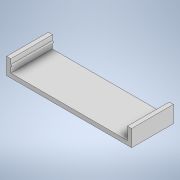
# Autodesk Inventor part: Houderpi
Saved by Autodesk Inventor 2021 (Build 250183000, 183)
## iProperties
Created: 2023-11-14
Part Number: Houderpi
Material: Generic
Document SubType Name: Modeling
Designer: Elias
Density: 1 g/cm^3
Appearance: Default
Author: Elias
Autodesk Inventor part; units mm, degrees
ref_plane "YZ Plane" through (0, 0, 0) normal (1, 0, 0) x (0, 1, 0)
ref_plane "XZ Plane" through (0, 0, 0) normal (0, 1, 0) x (-1, 0, 0)
ref_plane "XY Plane" through (0, 0, 0) normal (0, 0, 1) x (1, 0, 0)
sketch "Sketch1" plane through (0, 0, 0) normal (0, 0, 1) x (1, 0, 0)
  line L0 (0, 0) -> (60, 0)
  line L1 (60, 0) -> (60, 8)
  line L2 (60, 8) -> (0, 8)
  line L3 (0, 8) -> (0, 0)
  dimension "d0" = 60
  dimension "d3" = 8
  constraints: 8 end point, 2 parallel, 1 horizontal, 1 perpendicular
  measures "d0" distance of L2.end L1.end
  measures "d3" distance of L0.end L1.end
extrude "Extrusion1" add sketch "Sketch1" along normal blind 20
sketch "Sketch2" plane through (0, 0, 20) normal (0, 0, 1) x (1, 0, 0)
  line L0 (0, 0) -> (60, 0) projected
  line L1 (2, 2) -> (58, 2)
  line L2 (60, 0) -> (60, 8) projected
  line L3 (2, 2) -> (2, 8)
  line L4 (60, 8) -> (0, 8) projected
  line L5 (58, 2) -> (58, 8)
  line L6 (58, 8) -> (2, 8)
  line L7 (0, 4.6) -> (60, 4.6) construction
  dimension "d5" = 2
  dimension "d6" = 56
  dimension "d7" = 2
  dimension "d12" = 4.6
  constraints: 10 end point, 2 horizontal, 2 perpendicular, 2 point on line, 1 vertical
  measures "d5" distance between parallel lines of L1 L0
  measures "d6" distance of L1.start L1.end
  measures "d7" distance from line of L2 L1.end
  measures "d12" distance between parallel lines of L0 L7
extrude "Extrusion2" cut sketch "Sketch2" against normal blind 20
sketch "Sketch3" plane through (0, 0, 20) normal (0, 0, 1) x (1, 0, 0)
  line L0 (0, 8) -> (0, 0) construction
  line L1 (0, 4.6) -> (60, 4.6) construction
  line L2 (60, 0) -> (60, 8) construction
  line L3 (0, 0) -> (60, 0) construction
  line L4 (2, 2) -> (2, 8) construction
  arc A0 (2, 4.6) -> (2, 5.6) centre (2, 5.1) ccw
  line L5 (2, 5.6) -> (2, 4.6)
  line L6 (58, 2) -> (58, 8) projected
  arc A1 (58, 5.6) -> (58, 4.6) centre (58, 5.1) ccw
  line L7 (58, 5.6) -> (58, 4.6)
  dimension "d13" = 4.6
  dimension "d17" = 1
  dimension "d18" = 5.1
  dimension "d19" = 1
  dimension "d20" = 5.1
  constraints: 8 point on line, 6 end point, 4 point on circle, 2 centre point, 1 horizontal, 1 perpendicular, 1 vertical
  measures "d13" distance between parallel lines of L3 L1
  measures "d17" diameter of A0
  measures "d18" distance from line of L3 A0.centre
  measures "d19" diameter of A1
  measures "d20" distance from line of L3 A1.centre
extrude "Extrusion3" add sketch "Sketch3" against normal blind 20 contours L5 A0
body "Solid1"
